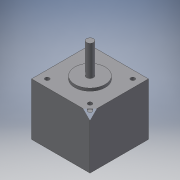
# Autodesk Inventor part: Part2
Saved by Autodesk Inventor 2016 (Build 200138000, 138)
## iProperties
Created: 2018-01-17
Part Number: Part2
Material: Generic
Document SubType Name: Modeling
Designer: student
Density: 1 g/cm^3
Appearance: Default
Author: student
Autodesk Inventor part; units mm, degrees
ref_plane "YZ Plane" through (0, 0, 0) normal (1, 0, 0) x (0, 1, 0)
ref_plane "XZ Plane" through (0, 0, 0) normal (0, 1, 0) x (-1, 0, 0)
ref_plane "XY Plane" through (0, 0, 0) normal (0, 0, 1) x (1, 0, 0)
sketch "Sketch1" plane through (0, 0, 0) normal (0, 1, 0) x (-1, 0, 0)
  line L0 (22.4859, 26.2748) -> (64.7859, 26.2748)
  line L1 (64.7859, 26.2748) -> (64.7859, -16.0252)
  line L2 (64.7859, -16.0252) -> (22.4859, -16.0252)
  line L3 (22.4859, -16.0252) -> (22.4859, 26.2748)
  point P0 (0, 0)
  dimension "d0" = 42.3
  dimension "d1" = 42.3
  constraints: 8 end point, 2 parallel, 1 horizontal, 1 perpendicular
  measures "d0" distance of L1.end L2.end
  measures "d1" distance of L0.end L1.end
extrude "Extrusion1" add sketch "Sketch1" along normal blind 38
sketch "Sketch2" plane through (0, 38, 0) normal (0, 1, 0) x (1, 0, 0)
  line L0 (-64.7859, -26.2748) -> (-22.4859, -26.2748) construction
  line L1 (-22.4859, -26.2748) -> (-22.4859, 16.0252) construction
  line L2 (-22.4859, 16.0252) -> (-64.7859, 16.0252) construction
  line L3 (-64.7859, 16.0252) -> (-64.7859, -26.2748) construction
  line L4 (-28.1359, -20.6248) -> (-59.1359, -20.6248) construction
  line L5 (-59.1359, -20.6248) -> (-59.1359, 10.3752) construction
  line L6 (-59.1359, 10.3752) -> (-28.1359, 10.3752) construction
  line L7 (-28.1359, 10.3752) -> (-28.1359, -20.6248) construction
  line L8 (-28.1359, -20.6248) -> (-59.1359, 10.3752) construction
  line L9 (-59.1359, -20.6248) -> (-28.1359, 10.3752) construction
  circle A0 centre (-59.1359, -20.6248) radius 1.5
  circle A1 centre (-59.1359, 10.3752) radius 1.5
  circle A2 centre (-28.1359, -20.6248) radius 1.5
  circle A3 centre (-28.1359, 10.3752) radius 1.5
  point P0 (0, 0)
  point P1 (-43.6359, -5.1248)
  dimension "d4" = 31
  dimension "d5" = 31
  dimension "d6" = 3
  dimension "d7" = 3
  dimension "d8" = 3
  dimension "d9" = 3
  constraints: 12 end point, 4 centre point, 4 coincident, 2 midpoint, 2 parallel, 1 horizontal, 1 perpendicular
  measures "d4" distance of L5.end L6.end
  measures "d5" distance of L4.end L5.end
  measures "d6" diameter of A0
  measures "d7" diameter of A1
  measures "d8" diameter of A2
  measures "d9" diameter of A3
extrude "Extrusion2" cut sketch "Sketch2" against normal blind 4.5
sketch "Sketch3" plane through (0, 38, 0) normal (0, 1, 0) x (1, 0, 0)
  circle A0 centre (-28.1359, -20.6248) radius 1.5 construction
  circle A1 centre (-59.1359, -20.6248) radius 1.5 construction
  circle A2 centre (-59.1359, 10.3752) radius 1.5 construction
  circle A3 centre (-28.1359, 10.3752) radius 1.5 construction
  line L0 (-64.7859, -26.2748) -> (-22.4859, -26.2748) construction
  line L1 (-22.4859, -26.2748) -> (-22.4859, 16.0252) construction
  line L2 (-22.4859, 16.0252) -> (-64.7859, 16.0252) construction
  line L3 (-64.7859, 16.0252) -> (-64.7859, -26.2748) construction
  circle A4 centre (-43.6359, -5.1248) radius 11
  point P0 (0, 0)
  dimension "d12" = 22
  constraints: 1 centre point
  measures "d12" diameter of A4
extrude "Extrusion3" add sketch "Sketch3" along normal blind 2
sketch "Sketch4" plane through (-43.6359, 40, 5.1248) normal (0, 1, 0) x (1, 0, 0)
  circle A0 centre (0, 0) radius 11 construction
  circle A1 centre (15.5, -15.5) radius 1.5 construction
  circle A2 centre (-15.5, -15.5) radius 1.5 construction
  circle A3 centre (-15.5, 15.5) radius 1.5 construction
  circle A4 centre (15.5, 15.5) radius 1.5 construction
  line L0 (-21.15, -21.15) -> (21.15, -21.15) construction
  line L1 (21.15, -21.15) -> (21.15, 21.15) construction
  line L2 (21.15, 21.15) -> (-21.15, 21.15) construction
  line L3 (-21.15, 21.15) -> (-21.15, -21.15) construction
  arc A5 (-2.4972, 0.1192) -> (-1.9972, 1.5038) centre (0, 0) ccw
  line L4 (-2.4972, 0.1192) -> (-1.9972, 1.5038)
  point P0 (43.6359, 5.1248)
  dimension "d15" = 5
  dimension "d16" = 0.5
  constraints: 2 end point, 2 point on circle, 1 centre point, 1 coincident
  measures "d15" diameter of A5
  measures "d16" horizontal distance of L4.start L4.end
extrude "Extrusion4" add sketch "Sketch4" along normal blind 22
body "Solid1"
